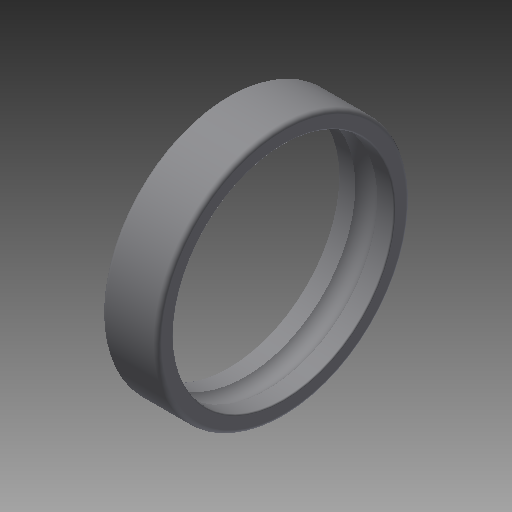
# Autodesk Inventor part: 6008_PART2
Saved by Autodesk Inventor 2018 (Build 220112000, 112)
## iProperties
Category: PARTsolutions
Company: SKF
Created: 2018-11-17
Part Number: 6008_PART2
Material: Generic
Catalog Web Link: www.cadenas.de
Description: -Deep groove ball bearings
Vendor: SKF
Document SubType Name: Modeling
Designer: psadmin
Manufacturer: SKF
Mass: 11.8876 g
Surface Area: 76.5014 cm^2
Volume: 11.8876 cm^3
Density: 1 g/cm^3
Appearance: PSOLRGB-175-175-175
PSOL_IDENT_0: {$CADENAS_DATA\23d-libs\skf\bearings_units_and_housings\ball_bearings\deep_groove_ball_bearings\bb1_
PSOL_IDENT_1: 001_101.prj},186 {VTYP=3D},{NB=6008_PART2},{LINA=6008_PART2},{NN=BB1_001_101_PART2},{NOPRJ=TRUE},{DA
PSOL_IDENT_2: TE=05.11.2018 07:58:23},{GEOMDATE=08.08.2018 12:16:40},{VERSION=},{LINEID=6500},{WBVAR=},{WBNUMERIC=
PSOL_IDENT_3: }  {NB=6008_PART2},{LINA=6008_PART2},{KT=DUMMY},{PRODUCTID=1050010008},{DESIGNATION=6008},{DD=40.00}
PSOL_IDENT_4: ,{D=68.000},{B=15.000},{C=0.000},{DD1=49.25},{DD2=0.0},{D1=0.00},{D2=61.10},{D3=0.00},{D4=0.000},{HH=
PSOL_IDENT_5: MIN},{BB=0.000},{FF=0.00},{R0MAX=MIN},{R0=MIN},{R12=1.10},{PITCH=54.00},{DW=7.938},{DDAMIN=44.600},{
PSOL_IDENT_6: DDAMAX=MIN},{DDBMIN=MIN},{DDBMAX=MIN},{DBMIN=MIN},{DAMAX=63.400},{BBAMIN=MIN},{CAMAX=MIN},{RAMAX=1.0
PSOL_IDENT_7: 00},{LOAD1=17.800},{LOAD2=11.000},{LOAD3=0.490},{SPEED1=22000},{SPEED2=14000},{KR=0.025},{F0=15.000}
PSOL_IDENT_8: ,{Z=12},{II=1},{MASS=0.192},{BEARING=6008},{RING=},{HELP=4.341},{HELP2=3.450},{DD1ALG=24.625},{YALG=
PSOL_IDENT_9: 24.625},{PITCH1=54.000},{DW1=7.938},{YALG1=29.659},{HALG1=4.341},{SH=24.625},{CU=1.412},{DESIGN=dgbb
PSOL_IDENT_10: 1},{HALG=4.625},{B1=0},{ALGO=1.000}
NT: Deep groove ball bearings
NB: 6008_PART2
NBSYN: $DESIGNATION._PART2
LINA: 6008_PART2
SUPPLIER: SKF
ARTICLENO: 6008_PART2
BOMINFO: 6008_PART2
CREATOR: CADENAS GmbH
Title: 6008_PART2
Author: Cadenas PARTsolutions
Comments: Deep groove ball bearings
Autodesk Inventor part; units mm, degrees
ref_plane "YZ Plane" through (0, 0, 0) normal (1, 0, 0) x (0, 1, 0)
ref_plane "XZ Plane" through (0, 0, 0) normal (0, 1, 0) x (-1, 0, 0)
ref_plane "XY Plane" through (0, 0, 0) normal (0, 0, 1) x (1, 0, 0)
sketch "Sketch_1" plane through (0, 0, 0) normal (0, 0, 1) x (1, 0, 0)
  line L0 (50, 0) -> (-50, 0)
  line L1 (0, 32.9) -> (0, 30.0257)
  arc A0 (0, 30.0257) -> (0.3667, 29.659) centre (0.3667, 30.0257) ccw
  line L2 (0.3667, 29.659) -> (4.5534, 29.659)
  arc A1 (10.4466, 29.659) -> (4.5534, 29.659) centre (7.5, 27) ccw
  line L3 (10.4466, 29.659) -> (14.6333, 29.659)
  arc A2 (14.6333, 29.659) -> (15, 30.0257) centre (14.6333, 30.0257) ccw
  line L4 (15, 30.0257) -> (15, 32.9)
  arc A3 (15, 32.9) -> (13.9, 34) centre (13.9, 32.9) ccw
  line L5 (13.9, 34) -> (1.1, 34)
  arc A4 (1.1, 34) -> (0, 32.9) centre (1.1, 32.9) ccw
  constraints: 12 end point, 10 point on circle, 5 centre point
revolve "Revolution1" add sketch "Sketch_1" angle 360 about axis through (50, 0, 0) along (1, 0, 0)
body "Solid1"
